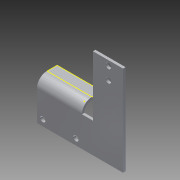
# Autodesk Inventor part: endstop 3
Saved by Autodesk Inventor 2013 (Build 170138000, 138)
## iProperties
Created: 2013-01-24
Part Number: endstop 3
Material: Aluminum 6061
Document SubType Name: Sheet Metal
Designer: Arpan
Density: 2.71 g/cm^3
Sheet Metal Rule: Default
Mass: 44.7583 g
Surface Area: 117.075 cm^2
Volume: 16.516 cm^3
Flat Pattern Width: 11.43 cm
Flat Pattern Length: 10.9144 cm
Flat Pattern Area: 124.751 cm^2
Sheet Metal Width: 4.500 in
Sheet Metal Length: 4.297 in
Sheet Metal Area: 19.337 in^2
Author: Arpan
Autodesk Inventor part; units mm, degrees
ref_plane "YZ Plane" through (0, 0, 0) normal (1, 0, 0) x (0, 1, 0)
ref_plane "XZ Plane" through (0, 0, 0) normal (0, 1, 0) x (-1, 0, 0)
ref_plane "XY Plane" through (0, 0, 0) normal (0, 0, 1) x (1, 0, 0)
sketch "Sketch1" plane through (0, 0, 0) normal (0, 0, 1) x (1, 0, 0)
  line L0 (0, 0) -> (-56.9976, 0)
  line L1 (-56.9976, 0) -> (-56.9976, 38.1)
  line L2 (-56.9976, 38.1) -> (0, 38.1)
  line L3 (0, 38.1) -> (0, 0)
  line L4 (0, 38.1) -> (-7.493, 38.1)
  line L5 (-7.493, 38.1) -> (-7.493, 8.1026)
  line L6 (-56.9976, 38.1) -> (-49.5046, 38.1)
  line L7 (-49.5046, 38.1) -> (-49.5046, 8.1026)
  dimension "d1" = 56.9976
  dimension "d2" = 38.1
  dimension "d3" = 7.493
  dimension "d4" = 29.9974
  dimension "d5" = 7.493
  measures "d1" distance of L0.start L0.end
  measures "d2" distance of L0.end L1.end
  measures "d3" distance of L2.end L4.end
  measures "d4" distance of L4.end L5.end
  measures "d5" distance of L1.end L6.end
extrude "Plate1" add sketch "Sketch1" along normal blind 3.175
sketch "Sketch2" plane through (0, 47.625, -9.525) normal (0, 1, 0) x (-1, 0, 0)
  line L0 (56.9976, 0) -> (0, 0)
  line L1 (0, 0) -> (0, -12.7)
  line L2 (0, -12.7) -> (56.9976, -12.7)
  line L3 (56.9976, -12.7) -> (56.9976, 0)
  constraints: 6 end point, 1 horizontal, 1 perpendicular, 1 vertical
edge flange "Flange1" height 25.4 angle 90 thickness 3.175 bend radius 9.525 thickness toward (0, 1, 0) relief straight relief width 3.175 relief depth 1.5875 corner gap 3.175 corner form 0 edges at (-53.2511, 38.1, 0) (-28.4988, 38.1, 0) (-3.7465, 38.1, 0) wall of the first edge with corners at (-56.9976, 47.625, -9.525) (0, 47.625, -9.525) (0, 47.625, -22.225) (-56.9976, 47.625, -22.225)
bend "Bend1"
corner "Corner1"
sketch "Sketch8" plane through (0, 0, 3.175) normal (0, 0, 1) x (1, 0, 0)
  circle A0 centre (-7.5, 7.9) radius 3.3 projected
  circle A1 centre (-49.5, 7.9) radius 3.3 projected
extrude "Cut1" cut sketch "Sketch8" against normal blind 3.175
sketch "Sketch9" plane through (-56.9976, 50.8, -22.225) normal (0, 1, 0) x (1, 0, 0)
  line L0 (0, -12.7) -> (56.9976, -12.7) projected
  line L1 (56.9976, 0) -> (56.9976, -12.7) projected
  line L2 (0, 0) -> (56.9976, 0) projected
  line L3 (0, -12.7) -> (0, 0) projected
  point P0 (56.9976, -22.225)
sketch "Sketch10" plane through (0, 0, 3.175) normal (1, 0, 0) x (0, 0, -1)
  line L0 (0, 38.1) -> (0, 0) projected
  line L1 (3.175, 0) -> (0, 0) projected
  line L2 (3.175, 0) -> (3.175, 38.1) projected
  line L3 (3.175, 38.1) -> (0, 38.1) projected
extrude "Extrusion1" add sketch "Sketch10" along normal blind 52.1462
sketch "Sketch13" plane through (0, 38.1, 3.175) normal (0, 1, 0) x (1, 0, 0)
  line L0 (0, 3.175) -> (0, 0) projected
  line L1 (0, 0) -> (52.1462, 0) projected
  line L2 (52.1462, 3.175) -> (52.1462, 0) projected
  line L3 (0, 3.175) -> (52.1462, 3.175) projected
extrude "Extrusion2" add sketch "Sketch13" along normal blind 76.2
sketch "Sketch14" plane through (0, 0, 0) normal (0, 0, -1) x (-1, 0, 0)
  circle A0 centre (-33.6026, 107.95) radius 3.3782 projected
  circle A1 centre (-33.6026, 92.075) radius 3.3782 projected
  point P0 (0, 0)
extrude "Cut4" cut sketch "Sketch14" against normal blind 3.175
sketch "Sketch15" plane through (0, 0, 3.175) normal (0, 0, 1) x (1, 0, 0)
  line L0 (0, 114.3) -> (52.1462, 114.3) projected
  line L1 (0, 38.1) -> (0, 114.3) projected
  line L2 (-56.9976, 38.1) -> (0, 38.1) projected
  line L3 (52.1462, 114.3) -> (14.0462, 114.3)
  line L4 (14.0462, 114.3) -> (14.0462, 38.1)
  line L5 (14.0462, 38.1) -> (0, 38.1)
  point P0 (0, 0)
  dimension "d31" = 38.1
  constraints: 6 end point, 1 collinear, 1 perpendicular, 1 point on line
  measures "d31" distance of L0.end L3.end
extrude "Cut5" cut sketch "Sketch15" against normal blind 3.175
equation "\"d19\" = Thickness"
equation "\"d29\" = Thickness"
equation "\"d32\" = Thickness"
equation "\"d9\" = BendReliefWidth"
equation "\"d10\" = BendReliefDepth"
equation "\"d11\" = MinimumRemnant"
equation "\"d12\" = BendRadius"
equation "\"d16\" = CornerReliefSize"
equation "\"d17\" = GapSize"
equation "\"d18\" = JacobiRadiusSize"
equation "\"BendRadius\" = Thickness"
equation "\"BendReliefWidth\" = Thickness"
equation "\"BendReliefDepth\" = 0.5 * Thickness"
equation "\"CornerReliefSize\" = 4 * Thickness"
equation "\"MinimumRemnant\" = 2 * Thickness"
equation "\"TransitionRadius\" = BendRadius"
equation "\"JacobiRadiusSize\" = BendRadius"
equation "\"GapSize\" = Thickness"
equation "\"d8\" = BendRadius"
equation "\"Thickness\" = 3.175"
body "Solid1"
